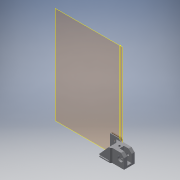
# Autodesk Inventor part: Ystartnew
Saved by Autodesk Inventor 2016 (Build 200138000, 138)
## iProperties
Created: 2016-07-16
Part Number: Ystartnew
Material: Generic
Document SubType Name: Modeling
Designer: Scott
Density: 1 g/cm^3
Appearance: Default
Author: Scott
Autodesk Inventor part; units mm, degrees
ref_plane "YZ Plane" through (0, 0, 0) normal (1, 0, 0) x (0, 1, 0)
ref_plane "XZ Plane" through (0, 0, 0) normal (0, 1, 0) x (-1, 0, 0)
ref_plane "Work Plane1" through (0, 0, 0) normal (0, 0, 1) x (1, 0, 0)
ref_plane "Work Plane2" through (127, 182.5, 0) normal (1, 0, 0) x (0, 1, 0)
sketch "Sketch1" plane through (127, 182.5, 0) normal (1, 0, 0) x (0, 1, 0)
  line L0 (0, -3.81) -> (-365, -3.81) projected
  line L1 (0, 0) -> (0, -3.81) projected
  line L2 (0, 0) -> (-365, 0) projected
  line L3 (-365, 0) -> (-365, -3.81) projected
  line L4 (-371.35, 459.74) -> (-371.35, 2.54) projected
  line L5 (-367.54, 2.54) -> (-371.35, 2.54) projected
  line L6 (-367.54, 459.74) -> (-367.54, 2.54) projected
  line L7 (-367.54, 459.74) -> (-371.35, 459.74) projected
  line L8 (-367.54, 46.355) -> (-363.73, 46.355)
  line L9 (-321.185, -3.81) -> (-321.185, -7.62)
  line L10 (-321.185, -7.62) -> (-375.16, -7.62)
  line L11 (-375.16, -7.62) -> (-375.16, 46.355)
  line L12 (-363.73, 46.355) -> (-363.73, 2.54)
  line L13 (-363.73, 2.54) -> (-321.185, 2.54)
  line L14 (-321.185, 2.54) -> (-321.185, 0)
  line L15 (-321.185, 0) -> (-365, 0)
  line L16 (-365, 0) -> (-365, -3.81)
  line L17 (-365, -3.81) -> (-321.185, -3.81)
  line L18 (-371.35, 46.355) -> (-371.35, 41.275)
  line L19 (-371.35, 41.275) -> (-371.35, 2.54)
  line L20 (-371.35, 2.54) -> (-367.54, 2.54)
  line L21 (-367.54, 2.54) -> (-367.54, 46.355)
  line L22 (-375.16, 46.355) -> (-371.35, 46.355)
  line L23 (-367.54, 46.355) -> (-363.73, 46.355)
  point P0 (-182.5, 0)
  point P1 (-326.265, 0)
  point P2 (-326.265, -3.81)
  point P3 (-367.54, 41.275)
  dimension "d2" = 3.81
  dimension "d4" = 3.81
  constraints: 32 end point, 7 collinear, 6 perpendicular, 5 point on line, 2 vertical, 1 parallel, 4 other
  measures "d2" distance of L8.start L8.end
  measures "d4" distance of L9.start L9.end
extrude "Extrusion1" add sketch "Sketch1" against normal blind 38.1 contours L9 L10 L11 L22 L4 L5 L6 L8 L12 L13 L14 L2 L3 L0
sketch "Sketch2" plane through (127, 182.5, 0) normal (1, 0, 0) x (0, 0, -1)
  line L0 (3.81, -365) -> (0, -365) projected
  line L1 (0, -365) -> (0, -321.185) projected
  line L2 (0, -321.185) -> (-2.54, -321.185) projected
  line L3 (-2.54, -321.185) -> (-2.54, -363.73) projected
  line L4 (-2.54, -363.73) -> (-46.355, -363.73) projected
  line L5 (-46.355, -363.73) -> (-46.355, -367.54) projected
  line L6 (-46.355, -367.54) -> (-2.54, -367.54) projected
  line L7 (-2.54, -367.54) -> (-2.54, -371.35) projected
  line L8 (-2.54, -371.35) -> (-46.355, -371.35) projected
  line L9 (-46.355, -371.35) -> (-46.355, -375.16) projected
  line L10 (-46.355, -375.16) -> (7.62, -375.16) projected
  line L11 (7.62, -375.16) -> (7.62, -321.185) projected
  line L12 (7.62, -321.185) -> (3.81, -321.185) projected
  line L13 (3.81, -321.185) -> (3.81, -365) projected
  line L14 (3.81, -321.185) -> (7.62, -321.185) projected
  line L15 (7.62, -375.16) -> (-46.355, -375.16) projected
  line L16 (7.62, -321.185) -> (-46.355, -321.185)
  line L17 (-46.355, -321.185) -> (-46.355, -375.16)
  line L18 (-46.355, -375.16) -> (7.62, -375.16)
  line L19 (7.62, -375.16) -> (7.62, -321.185)
  point P0 (0, -182.5)
  constraints: 8 end point, 2 parallel, 1 horizontal, 1 perpendicular
extrude "Extrusion2" add sketch "Sketch2" along normal blind 5.08
sketch "Sketch3" plane through (88.9, -138.685, -3.81) normal (0, 1, 0) x (1, 0, 0)
  line L0 (38.1, -3.81) -> (0, -3.81) projected
  line L1 (0, -6.35) -> (0, -3.81) projected
  line L2 (38.1, -6.35) -> (0, -6.35) projected
  line L3 (38.1, -6.35) -> (38.1, -50.165) projected
  line L4 (38.1, -50.165) -> (43.18, -50.165) projected
  line L5 (43.18, 3.81) -> (43.18, -50.165) projected
  line L6 (0, 3.81) -> (43.18, 3.81) projected
  line L7 (0, 0) -> (0, 3.81) projected
  line L8 (38.1, 0) -> (0, 0) projected
  line L9 (38.1, 0) -> (38.1, -3.81) projected
  line L10 (43.18, -50.165) -> (43.18, 3.81) projected
  line L11 (43.18, -23.1775) -> (55.88, -23.1775)
  circle A0 centre (55.88, -23.1775) radius 4
  line L12 (55.88, -27.1775) -> (55.88, -32.2575)
  line L13 (55.88, -19.1775) -> (55.88, -14.0975)
  line L14 (59.88, -23.1775) -> (64.96, -23.1775)
  line L15 (43.18, -14.0975) -> (64.96, -14.0975)
  line L16 (64.96, -14.0975) -> (64.96, -32.2575)
  line L17 (64.96, -32.2575) -> (43.18, -32.2575)
  line L18 (43.18, -32.2575) -> (43.18, -14.0975)
  point P0 (-88.9, -3.81)
  dimension "d9" = 12.7
  dimension "d10" = 8
  dimension "d11" = 5.08
  dimension "d12" = 5.08
  dimension "d13" = 5.08
  constraints: 16 end point, 3 horizontal, 3 point on circle, 2 parallel, 2 vertical, 1 centre point, 1 coincident, 1 midpoint, 1 perpendicular, 1 point on line
  measures "d9" distance of L11.start L11.end
  measures "d10" diameter of A0
  measures "d11" distance of L12.start L12.end
  measures "d12" distance of L13.start L13.end
  measures "d13" distance of L14.start L14.end
extrude "Extrusion3" add sketch "Sketch3" against normal up to surface (53.975 mm away) contours L15 L13 A0 L11 L5 | L5 L11 A0 L12 L17 | L15 L16 L14 A0 L13 | L12 A0 L14 L16 L17
sketch "Sketch4" plane through (132.08, -138.685, 28.4475) normal (0, 0, 1) x (1, 0, 0)
  line L0 (0, -53.975) -> (21.78, -53.975) projected
  line L1 (21.78, 0) -> (21.78, -53.975) projected
  line L2 (0, 0) -> (21.78, 0) projected
  line L3 (0, -53.975) -> (0, 0) projected
  line L4 (0, -53.975) -> (0, 0) projected
  line L5 (21.78, 0) -> (21.78, -53.975) projected
  line L6 (0, -45.966) -> (21.78, -45.966)
  line L7 (21.78, -45.966) -> (21.78, -26.916)
  line L8 (21.78, -26.916) -> (0, -26.916)
  line L9 (0, -26.916) -> (0, -45.966)
  line L10 (21.78, -45.966) -> (53.53, -45.966)
  line L11 (53.53, -45.966) -> (53.53, 0)
  line L12 (53.53, 0) -> (21.78, 0)
  line L13 (21.78, 0) -> (21.78, -45.966)
  circle A0 centre (37.655, -22.983) radius 11
  point P0 (-132.08, 138.685)
  dimension "d16" = 19.05
  dimension "d17" = 31.75
  dimension "d18" = 22
  constraints: 16 end point, 4 parallel, 2 horizontal, 2 perpendicular, 2 point on line, 1 centre point
  measures "d16" distance of L7.end L6.end
  measures "d17" distance of L12.end L11.end
  measures "d18" diameter of A0
extrude "Extrusion4" add sketch "Sketch4" along normal blind 5.08 contours L3 L8 L1 L6 | L1 L12 L11 L10 | L3 L2 L1 L8
sketch "Sketch5" plane through (153.86, -138.685, 10.2875) normal (0, 0, -1) x (-1, 0, 0)
  circle A0 centre (-15.875, -22.983) radius 11 projected
  line L0 (21.78, -45.966) -> (-31.75, -45.966) projected
  line L1 (-31.75, -45.966) -> (-31.75, 0) projected
  line L2 (-31.75, 0) -> (21.78, 0) projected
  line L3 (21.78, -45.966) -> (21.78, 0) projected
  point P0 (153.86, 138.685)
extrude "Extrusion5" add sketch "Sketch5" along normal blind 5.08
sketch "Sketch6" plane through (132.08, -138.685, 33.5275) normal (0, 0, 1) x (1, 0, 0)
  circle A0 centre (37.655, -22.983) radius 11 projected
  line L0 (0, -45.966) -> (53.53, -45.966) projected
  line L1 (53.53, -45.966) -> (53.53, 0) projected
  line L2 (53.53, 0) -> (0, 0) projected
  line L3 (0, -45.966) -> (0, 0) projected
  point P0 (-132.08, 138.685)
extrude "Extrusion6" add sketch "Sketch6" along normal blind 8
sketch "Sketch7" plane through (132.08, -138.685, 28.4475) normal (0, 0, -1) x (-1, 0, 0)
  line L0 (-53.53, -45.966) -> (-53.53, 0) projected
  circle A0 centre (-37.655, -22.983) radius 11 projected
  line L1 (0, -45.966) -> (-53.53, -45.966) projected
  line L2 (-53.53, -45.966) -> (-53.53, 0) projected
  line L3 (-53.53, 0) -> (0, 0) projected
  line L4 (0, -45.966) -> (0, 0) projected
  circle A1 centre (-37.655, -22.983) radius 5
  point P0 (132.08, 138.685)
  dimension "d25" = 10
  constraints: 1 centre point, 1 coincident
  measures "d25" diameter of A1
extrude "Extrusion7" add sketch "Sketch7" against normal blind 5.08 contours A0
chamfer "Chamfer1" distance 4.7625 angle 45 1 edges at (132.08, -161.668, 41.5275)
sketch "Sketch8" plane through (153.86, -138.685, 10.2875) normal (0, 0, 1) x (1, 0, 0)
  circle A0 centre (15.875, -22.983) radius 5 projected
  circle A1 centre (15.875, -22.983) radius 11 projected
  point P0 (-153.86, 138.685)
extrude "Extrusion8" add sketch "Sketch8" against normal blind 5.08
sketch "Sketch9" plane through (153.86, -138.685, 5.2075) normal (0, 0, -1) x (-1, 0, 0)
  circle A0 centre (-15.875, -22.983) radius 5 projected
  line L0 (-31.75, -45.966) -> (21.78, -45.966) projected
  line L1 (21.78, 0) -> (21.78, -45.966) projected
  line L2 (21.78, 0) -> (-31.75, 0) projected
  line L3 (-31.75, 0) -> (-31.75, -45.966) projected
  circle A1 centre (-15.875, -22.983) radius 11 projected
  point P0 (153.86, 138.685)
extrude "Extrusion9" add sketch "Sketch9" along normal blind 7 contours L3 L2 L1 L0
chamfer "Chamfer2" distance 4.7625 angle 45 1 edges at (132.08, -161.668, -1.7925)
sketch "Sketch10" plane through (153.86, -184.651, 28.4475) normal (0, -1, 0) x (1, 0, 0)
  line L0 (4.875, -23.24) -> (26.875, -23.24) projected
  line L1 (-21.78, -18.16) -> (0, -18.16) projected
  line L2 (-21.78, -35.0025) -> (-21.78, -18.16) projected
  line L3 (-17.0175, -30.24) -> (-21.78, -35.0025) projected
  line L4 (31.75, -30.24) -> (-17.0175, -30.24) projected
  line L5 (31.75, -18.16) -> (31.75, -30.24) projected
  line L6 (0, -18.16) -> (31.75, -18.16) projected
  line L7 (4.875, 5.08) -> (26.875, 5.08) projected
  line L8 (0, 0) -> (-21.78, 0) projected
  line L9 (0, 0) -> (31.75, 0) projected
  line L10 (31.75, 0) -> (31.75, 13.08) projected
  line L11 (-17.0175, 13.08) -> (31.75, 13.08) projected
  line L12 (-21.78, 17.8425) -> (-17.0175, 13.08) projected
  line L13 (-21.78, 0) -> (-21.78, 17.8425) projected
  line L14 (0, 0) -> (31.75, 0) projected
  line L15 (31.75, -30.24) -> (0, -30.24)
  line L16 (0, -30.24) -> (0, 0)
  line L17 (0, 0) -> (31.75, 0)
  line L18 (31.75, 0) -> (31.75, -30.24)
  point P0 (-153.86, -28.4475)
  constraints: 8 end point, 2 parallel, 1 horizontal, 1 perpendicular
extrude "Extrusion10" add sketch "Sketch10" along normal up to surface (8.009 mm away)
sketch "Sketch11" plane through (88.9, -185.04, 46.355) normal (0, 0, 1) x (1, 0, 0)
  line L0 (38.1, 3.81) -> (0, 3.81) projected
  line L1 (0, 0) -> (0, 3.81) projected
  line L2 (38.1, 0) -> (0, 0) projected
  line L3 (38.1, 0) -> (38.1, -3.81) projected
  line L4 (38.1, -3.81) -> (0, -3.81) projected
  line L5 (0, -7.62) -> (0, -3.81) projected
  line L6 (0, -7.62) -> (43.18, -7.62) projected
  line L7 (43.18, 46.355) -> (43.18, -7.62) projected
  line L8 (38.1, 46.355) -> (43.18, 46.355) projected
  line L9 (38.1, 46.355) -> (38.1, 3.81) projected
  line L10 (0, 0) -> (0, 3.81) projected
  line L11 (38.1, 46.355) -> (0, 3.81)
  line L12 (38.1, 3.81) -> (0, 3.81) projected
  line L13 (0, 3.81) -> (38.1, 3.81)
  line L14 (38.1, 3.81) -> (38.1, 46.355)
  point P0 (-88.9, 185.04)
  constraints: 6 end point, 1 collinear
extrude "Extrusion11" add sketch "Sketch11" against normal blind 2.54 contours L0 L11 L9
sketch "Sketch12" plane through (88.9, -181.23, 2.54) normal (0, 0, 1) x (1, 0, 0)
  circle A0 centre (17.78, 13.97) radius 3.175 projected
  circle A1 centre (17.78, 34.29) radius 3.175 projected
  circle A2 centre (17.78, 13.97) radius 3.175 projected
  point P0 (-88.9, 181.23)
extrude "Extrusion12" cut sketch "Sketch12" against normal blind 45.4025
sketch "Sketch13" plane through (88.9, -181.23, 2.54) normal (0, 1, 0) x (1, 0, 0)
  circle A0 centre (17.78, -15.24) radius 3.175 projected
  circle A1 centre (17.78, -35.56) radius 3.175 projected
  point P0 (-88.9, 2.54)
extrude "Extrusion13" cut sketch "Sketch13" along normal mid plane 45.4025
chamfer "Chamfer3" distance 12.7 angle 45 2 edges at (127, -159.9575, 2.54) (127, -181.23, 23.1775)
chamfer "Chamfer4" distance 12.7 angle 45 2 edges at (185.61, -138.685, 4.2475) (185.61, -138.685, 34.9875)
sketch "Sketch14" plane through (88.9, -192.66, -7.62) normal (0, 0, -1) x (-1, 0, 0)
  circle A0 centre (-17.78, 25.4) radius 3.175 projected
  circle A1 centre (-17.78, 45.72) radius 3.175 projected
  line L0 (0, 0) -> (-43.18, 0) projected
  line L1 (0, 53.975) -> (0, 0) projected
  line L2 (0, 53.975) -> (-43.18, 53.975) projected
  line L3 (-43.18, 0) -> (-43.18, 53.975) projected
  line L4 (-43.18, 53.975) -> (-34.1997, 62.9553)
  line L5 (-43.18, 53.975) -> (-30.48, 53.975) construction
  line L6 (-34.1997, 62.9553) -> (0, 62.9553)
  line L7 (-25.4, 53.975) -> (0, 53.975) projected
  line L8 (0, 62.9553) -> (0, 53.975)
  line L9 (-47.9425, 53.975) -> (-43.18, 53.975) projected
  line L10 (-43.18, 53.975) -> (0, 53.975)
  point P0 (88.9, 192.66)
  dimension "d52" = 12.7
  dimension "d53" = 45
  constraints: 10 end point, 2 horizontal, 1 collinear, 1 equal length, 1 perpendicular
  measures "d52" distance of L2.end L4.end
  measures "d53" angle of L5 L4
ref_plane "Work Plane3" through (-127, -182.5, -3.81) normal (0, 0, -1) x (0, 1, 0)
extrude "Extrusion14" add sketch "Sketch14" against normal up to surface (3.81 mm away) contours L2 L4 L6 L8
sketch "Sketch15" plane through (88.9, -182.5, 0) normal (0, 0, -1) x (-1, 0, 0)
  line L0 (-43.18, 43.815) -> (-34.1997, 52.7953) projected
  line L1 (-34.1997, 52.7953) -> (0, 52.7953) projected
  line L2 (-25.4, 43.815) -> (0, 43.815) projected
  line L3 (-38.1, 43.815) -> (-25.4, 43.815) projected
  line L4 (-38.1, 43.815) -> (-43.18, 43.815) projected
  line L5 (0, 0) -> (0, 52.7953) projected
  point P0 (88.9, 182.5)
extrude "Extrusion15" add sketch "Sketch15" against normal up to surface (2.54 mm away)
body "Solid1"
